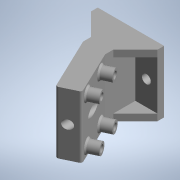
# Autodesk Inventor part: ir_camera_mount
Saved by Autodesk Inventor 2022 (Build 260153000, 153)
## iProperties
Part Number: ir_camera_mount
Material: Allgemein
Document SubType Name: Modellieren
Designer: Niclas
Appearance: Vorgabe
Author: Niclas
Autodesk Inventor part; units mm, degrees
ref_plane "YZ-Ebene" through (0, 0, 0) normal (1, 0, 0) x (0, 1, 0)
ref_plane "XZ-Ebene" through (0, 0, 0) normal (0, 1, 0) x (-1, 0, 0)
ref_plane "XY-Ebene" through (0, 0, 0) normal (0, 0, 1) x (1, 0, 0)
sketch "Skizze1" plane through (0, 0, 0) normal (0, 1, 0) x (-1, 0, 0)
  line L0 (-0.8169, 1.8861) -> (9.1831, 1.8861)
  line L1 (9.1831, 1.8861) -> (9.1831, -14.7439)
  line L2 (9.1831, -14.7439) -> (-0.8169, -14.7439)
  line L3 (-0.8169, -14.7439) -> (-0.8169, 1.8861)
  line L4 (-0.8169, 1.8861) -> (-10.2882, 21.743)
  line L5 (9.1831, 14.3218) -> (9.1831, 1.8861)
  line L6 (9.1831, 1.8861) -> (-2.1416, 25.6287)
  line L7 (-2.1416, 25.6287) -> (-10.2882, 21.743)
  point P0 (-5.5526, 11.8145)
  point P1 (9.1831, -3.6782)
  dimension "d23" = 154.5
  dimension "d24" = 10
  dimension "d25" = 22
  dimension "d26" = 16.63
  dimension "d27" = 9.9284
  constraints: 16 end point, 2 parallel, 2 perpendicular, 1 horizontal, 1 midpoint, 1 vertical
  measures "d23" angle of L3 L4
  measures "d24" distance of L1.end L2.end
  measures "d25" distance of L0.start L4.end
  measures "d26" distance of L2.end L0.start
  measures "d27" distance from line of L0 point (-5.553, 11.815)
extrude "Extrusion3" add sketch "Skizze1" along normal blind 28
sketch "Skizze4" plane through (0.8169, 0, 1.8861) normal (0.9026, 0, -0.4305) x (-0.4305, 0, -0.9026)
  circle A0 centre (-4.65, 24.16) radius 2.5
  circle A1 centre (-4.65, 3.84) radius 2.5
  circle A2 centre (-17.35, 3.84) radius 2.5
  circle A3 centre (-17.35, 24.16) radius 2.5
  line L0 (-22, 28) -> (0, 28) projected
  line L1 (-22, 0) -> (-22, 28) projected
  line L2 (0, 0) -> (0, 28) projected
  circle A4 centre (-4.65, 24.16) radius 1.5
  circle A5 centre (-4.65, 3.84) radius 1.5
  circle A6 centre (-17.35, 3.84) radius 1.5
  circle A7 centre (-17.35, 24.16) radius 1.5
  point P0 (2.0541, 0)
  dimension "d35" = 5
  dimension "d36" = 5
  dimension "d37" = 5
  dimension "d38" = 5
  dimension "d39" = 20.32
  dimension "d40" = 20.32
  dimension "d41" = 12.7
  dimension "d42" = 12.7
  dimension "d43" = 3.84
  dimension "d45" = 4.65
  dimension "d46" = 4.65
  dimension "d47" = 3.84
  dimension "d48" = 3
  dimension "d49" = 3
  dimension "d50" = 3
  dimension "d51" = 3
  constraints: 8 centre point, 4 coincident
  measures "d35" diameter of A0
  measures "d36" diameter of A1
  measures "d37" diameter of A2
  measures "d38" diameter of A3
  measures "d39" distance of A1.centre A0.centre
  measures "d40" distance of A2.centre A3.centre
  measures "d41" distance of A2.centre A1.centre
  measures "d42" distance of A3.centre A0.centre
  measures "d43" distance from line of L0 A0.centre
  measures "d45" distance from line of L2 A0.centre
  measures "d46" distance from line of L2 A1.centre
  measures "d47" distance from line of L0 A3.centre
  measures "d48" diameter of A4
  measures "d49" diameter of A7
  measures "d50" diameter of A6
  measures "d51" diameter of A5
extrude "Extrusion4" add sketch "Skizze4" along normal blind 5
extrude "Extrusion5" cut sketch "Skizze4" against normal blind 10 contours A4 | A5 | A6 | A7
sketch "Skizze6" plane through (-9.1831, 0, -14.7439) normal (-1, 0, 0) x (0, 0, 1)
  line L0 (0, 0) -> (16.63, 0) projected
  line L1 (0, 28) -> (16.63, 28) projected
  line L2 (0, 0) -> (3, 0)
  line L3 (3, 0) -> (3, 28)
  line L4 (3, 28) -> (0, 28)
  line L5 (0, 28) -> (0, 0)
  point P0 (14.7439, 0)
  point P1 (36.0154, 0)
  point P2 (36.0154, 28)
  point P3 (3, 0)
  dimension "d56" = 3
  constraints: 8 end point, 2 parallel, 1 horizontal, 1 perpendicular, 1 point on line
  measures "d56" distance of L4.end L3.end
extrude "Extrusion6" add sketch "Skizze6" along normal blind 10
sketch "Skizze7" plane through (0.8169, 0, 1.8861) normal (1, 0, 0) x (0, 0, -1)
  line L0 (16.63, 0) -> (16.63, 28) projected
  line L1 (0, 0) -> (16.63, 0) projected
  line L2 (16.63, 28) -> (13.63, 28)
  line L3 (13.63, 28) -> (13.63, 0)
  line L4 (13.63, 0) -> (16.63, 0)
  line L5 (16.63, 0) -> (16.63, 28)
  point P0 (1.8861, 0)
  dimension "d59" = 3
  constraints: 8 end point, 2 parallel, 1 horizontal, 1 perpendicular, 1 point on line
  measures "d59" distance of L4.end L3.end
extrude "Extrusion7" add sketch "Skizze7" along normal blind 10
sketch "Skizze8" plane through (0, 0, 0) normal (0, -1, 0) x (1, 0, 0)
  line L0 (0.8169, -11.7439) -> (10.8169, -11.7439) projected
  line L1 (10.8169, -11.7439) -> (0.8148, -1.7417)
  line L2 (10.8169, -11.7439) -> (24.9621, -11.7439) construction
  line L3 (-9.1831, -11.7439) -> (-19.1831, -11.7439) projected
  line L4 (-19.1831, -11.7439) -> (-9.1831, -1.7417)
  line L5 (-9.1831, -11.7439) -> (-9.1831, 1.8861) projected
  line L6 (10.8169, -14.7439) -> (10.8169, -11.7439) projected
  line L7 (10.8169, -11.7439) -> (-19.1831, -11.7439)
  line L8 (-9.1831, -1.7417) -> (0.8148, -1.7417)
  point P0 (0, 0)
  point P1 (-9.1831, 3.2715)
  point P2 (-9.1831, -11.7439)
  dimension "d62" = 135
  constraints: 10 end point, 1 equal length, 1 horizontal, 1 parallel, 1 point on line
  measures "d62" angle of L2 L1
extrude "Extrusion8" add sketch "Skizze8" against normal blind 3
sketch "Skizze9" plane through (0, 28, 0) normal (0, 1, 0) x (1, 0, 0)
  line L0 (-9.1831, 11.7439) -> (-19.1831, 11.7439) projected
  line L1 (-19.1831, 11.7439) -> (-9.1831, 1.7417)
  line L2 (-9.1831, 1.7417) -> (0.8169, 1.7417)
  line L3 (0.8169, -1.8861) -> (0.8169, 11.7439) projected
  line L4 (10.8169, 14.7439) -> (10.8169, 11.7439) projected
  line L5 (10.8169, 11.7439) -> (0.8169, 1.7417)
  line L6 (-19.1831, 11.7439) -> (10.8169, 11.7439)
  point P0 (0, 0)
  point P1 (-9.1831, 11.7439)
  constraints: 8 end point, 1 horizontal, 1 parallel, 1 point on line
extrude "Extrusion9" add sketch "Skizze9" against normal blind 3
sketch "Skizze10" plane through (-19.1831, 0, -14.7439) normal (0, 0, -1) x (-1, 0, 0)
  circle A0 centre (-5, 14) radius 2
  circle A1 centre (-25, 14) radius 2
  line L0 (0, 28) -> (0, 0) projected
  line L1 (-30, 0) -> (-30, 28) projected
  line L2 (0, 0) -> (-30, 0) projected
  point P0 (-19.1831, 0)
  dimension "d67" = 4
  dimension "d68" = 4
  dimension "d69" = 5
  dimension "d70" = 5
  dimension "d71" = 14
  dimension "d72" = 14
  constraints: 2 centre point
  measures "d67" diameter of A0
  measures "d68" diameter of A1
  measures "d69" distance from line of L0 A0.centre
  measures "d70" distance from line of L1 A1.centre
  measures "d71" distance from line of L2 A0.centre
  measures "d72" distance from line of L2 A1.centre
extrude "Extrusion10" cut sketch "Skizze10" against normal blind 50
sketch "Skizze11" plane through (0, 28, 0) normal (0, 1, 0) x (1, 0, 0)
  line L0 (10.8169, 14.7439) -> (10.8169, 11.7439) projected
  line L1 (-19.1831, 14.7439) -> (10.8169, 14.7439) projected
  line L2 (-19.1831, 11.7439) -> (-19.1831, 14.7439) projected
  line L3 (-19.1831, 11.7439) -> (-9.1831, 1.7417) projected
  line L4 (-9.1831, 1.7417) -> (-9.1831, -1.8861) projected
  line L5 (-9.1831, -1.8861) -> (2.1416, -25.6287) projected
  line L6 (2.1416, -25.6287) -> (10.2882, -21.743) projected
  line L7 (10.2882, -21.743) -> (0.8169, -1.8861) projected
  line L8 (0.8169, -1.8861) -> (0.8169, 1.7417) projected
  line L9 (0.8169, 1.7417) -> (10.8169, 11.7439) projected
  line L10 (-9.1831, 1.7417) -> (-9.1831, -1.8861) projected
  line L11 (-9.1831, -1.8861) -> (2.1416, -25.6287) projected
  line L12 (-9.1831, 1.7417) -> (-9.1831, -1.6598)
  line L13 (-9.0856, -2.0903) -> (1.7111, -24.7261)
  line L14 (2.1416, -25.6287) -> (10.2882, -21.743) projected
  line L15 (3.0442, -25.1982) -> (9.3856, -22.1735)
  line L16 (0.8169, -1.8861) -> (0.8169, 1.7417) projected
  line L17 (0.8169, 19.7417) -> (0.8169, -1.6598)
  line L18 (0.9144, -2.0903) -> (9.8577, -20.8404)
  arc A0 (-9.1831, -1.6598) -> (-9.0856, -2.0903) centre (-8.1831, -1.6598) ccw
  arc A1 (1.7111, -24.7261) -> (3.0442, -25.1982) centre (2.6137, -24.2956) ccw
  arc A2 (9.3856, -22.1735) -> (9.8577, -20.8404) centre (8.9551, -21.2709) ccw
  arc A3 (0.8169, -1.6598) -> (0.9144, -2.0903) centre (1.8169, -1.6598) ccw
  point P0 (0, 0)
  point P1 (9.3856, -22.1735)
  point P2 (3.0442, -25.1982)
  point P3 (1.7111, -24.7261)
  point P4 (-9.1831, -1.6598)
  point P5 (0.9144, -2.0903)
  point P6 (0.8169, -1.6598)
  dimension "d75" = 1
  dimension "d76" = 1
  constraints: 10 end point, 9 point on line, 8 point on circle, 8 tangent, 4 centre point, 4 collinear, 2 equal radius, 1 vertical
  measures "d75" radius of A0
  measures "d76" radius of A3
extrude "Extrusion11" cut sketch "Skizze11" against normal blind 30 contours L7 L6 A2 | A0 L5 L4 | L6 L5 A1
extrude "Extrusion12" add sketch "Skizze11" against normal blind 28 contours A3 L7 L8
chamfer "Fase3" distance 0.6 angle 45 1 edges at (9.3626, 24.16, 19.8024)
chamfer "Fase4" distance 0.6 angle 45 1 edges at (9.3626, 3.84, 19.8024)
chamfer "Fase5" distance 0.6 angle 45 2 edges at (3.8951, 24.16, 8.3396) (3.8951, 3.84, 8.3396)
